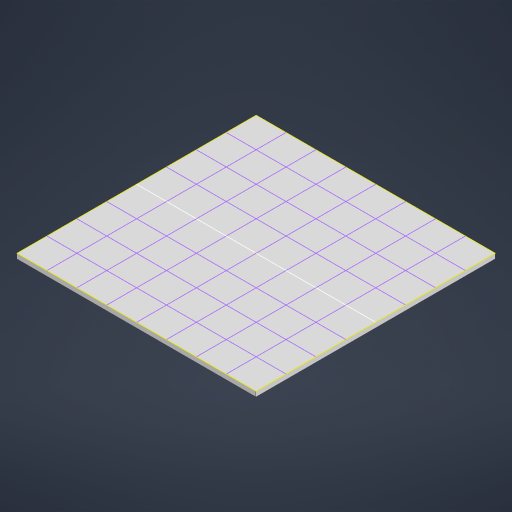
# Autodesk Inventor part: chessboard
Saved by Autodesk Inventor 2023 (Build 270158000, 158)
## iProperties
Created: 2023-11-06
Part Number: chessboard
Material: Generic
Document SubType Name: Modeling
Designer: hrush
Density: 1 g/cm^3
Appearance: Default
Author: hrush
Autodesk Inventor part; units mm, degrees
ref_plane "YZ Plane" through (0, 0, 0) normal (1, 0, 0) x (0, 1, 0)
ref_plane "XZ Plane" through (0, 0, 0) normal (0, 1, 0) x (-1, 0, 0)
ref_plane "XY Plane" through (0, 0, 0) normal (0, 0, 1) x (1, 0, 0)
sketch "Sketch1" plane through (0, 0, 0) normal (0, 1, 0) x (-1, 0, 0)
  line L0 (-120, 120) -> (120, 120)
  line L1 (120, 120) -> (120, -120)
  line L2 (120, -120) -> (-120, -120)
  line L3 (-120, -120) -> (-120, 120)
  line L4 (-120, 120) -> (120, -120) construction
  line L5 (120, 120) -> (-120, -120) construction
  point P0 (0, 0)
  dimension "d0" = 240
  dimension "d1" = 240
  constraints: 12 end point, 2 midpoint, 2 parallel, 1 horizontal, 1 perpendicular
  measures "d0" distance of L1.end L2.end
  measures "d1" distance of L0.end L1.end
extrude "Extrusion1" add sketch "Sketch1" along normal blind 5
sketch "Sketch2" plane through (0, 5, 0) normal (0, 1, 0) x (1, 0, 0)
  line L0 (-120, 120) -> (-120, -120) projected
  line L1 (-120, 0) -> (120, 0)
  line L2 (120, -120) -> (120, 120) projected
  line L3 (-120, -60) -> (120, -60)
  line L4 (-120, 60) -> (120, 60)
  line L5 (-120, -90) -> (120, -90)
  line L6 (-120, -30) -> (120, -30)
  line L7 (-120, 30) -> (120, 30)
  line L8 (-120, 90) -> (120, 90)
  line L9 (0, -120) -> (0, 120)
  line L10 (120, 120) -> (-120, 120) projected
  line L11 (-60, -120) -> (-60, 120)
  line L12 (-120, -120) -> (120, -120) projected
  line L13 (-90, -120) -> (-90, 120)
  line L14 (-30, -120) -> (-30, 120)
  line L15 (30, -120) -> (30, 120)
  line L16 (60, -120) -> (60, 120)
  line L17 (90, -120) -> (90, 120)
  point P0 (0, 0)
  constraints: 28 end point, 10 point on line, 9 perpendicular, 3 midpoint, 2 parallel, 1 horizontal
body "Solid1"
